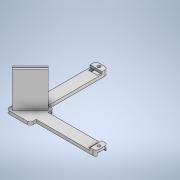
# Autodesk Inventor part: beamsplitter main
Saved by Autodesk Inventor 2022 (Build 260153000, 153)
## iProperties
Created: 2022-07-06
Part Number: beamsplitter main
Material: Generic
Document SubType Name: Modeling
Designer: Eli
Density: 1 g/cm^3
Appearance: Default
Author: Eli
Autodesk Inventor part; units mm, degrees
ref_plane "YZ Plane" through (0, 0, 0) normal (1, 0, 0) x (0, 1, 0)
ref_plane "XZ Plane" through (0, 0, 0) normal (0, 1, 0) x (-1, 0, 0)
sketch "Sketch1" plane through (0, 0, 0) normal (0, 1, 0) x (-1, 0, 0)
  line L0 (-6.35, 0) -> (-44.45, 0)
  line L1 (0, -44.45) -> (0, -6.35)
  line L2 (-38.1, -50.8) -> (-38.1, -171.45)
  line L3 (-31.75, -177.8) -> (-19.05, -177.8)
  line L4 (-12.7, -171.45) -> (-12.7, -50.8)
  line L5 (-25.4, 0) -> (-25.4, -50.8) construction
  line L6 (-44.45, -50.8) -> (-25.4, -50.8)
  line L7 (-12.7, -50.8) -> (-6.35, -50.8)
  line L8 (0, 0) -> (-50.8, -50.8) construction
  line L9 (-50.8, -38.1) -> (-171.45, -38.1)
  line L10 (-177.8, -31.75) -> (-177.8, -19.05)
  line L11 (-171.45, -12.7) -> (-50.8, -12.7)
  line L12 (-50.8, -6.35) -> (-50.8, -12.7)
  line L13 (-50.8, -38.1) -> (-50.8, -44.45)
  arc A0 (-50.8, -44.45) -> (-44.45, -50.8) centre (-44.45, -44.45) ccw
  arc A1 (-6.35, -50.8) -> (0, -44.45) centre (-6.35, -44.45) ccw
  arc A2 (0, -6.35) -> (-6.35, 0) centre (-6.35, -6.35) ccw
  arc A3 (-44.45, 0) -> (-50.8, -6.35) centre (-44.45, -6.35) ccw
  arc A4 (-19.05, -177.8) -> (-12.7, -171.45) centre (-19.05, -171.45) ccw
  arc A5 (-38.1, -171.45) -> (-31.75, -177.8) centre (-31.75, -171.45) ccw
  arc A6 (-171.45, -12.7) -> (-177.8, -19.05) centre (-171.45, -19.05) ccw
  arc A7 (-177.8, -31.75) -> (-171.45, -38.1) centre (-171.45, -31.75) ccw
  point P0 (-50.8, 0)
  point P1 (0, -50.8)
  point P2 (-38.1, -177.8)
  point P3 (-12.7, -177.8)
  point P4 (-177.8, -38.1)
  point P5 (-177.8, -12.7)
  dimension "d0" = 50.8
  dimension "d1" = 50.8
  dimension "d2" = 25.4
  dimension "d3" = 127
  dimension "d4" = 6.35
  dimension "d5" = 6.35
  dimension "d6" = 6.35
  constraints: 28 end point, 16 point on circle, 16 point on line, 16 tangent, 8 centre point, 5 equal radius, 5 parallel, 4 symmetric about line, 2 horizontal, 2 perpendicular, 1 midpoint, 1 vertical, 1 other
  measures "d0" distance of point (0, -50.8) L8.start
  measures "d1" distance of L8.start point (-50.8, 0)
  measures "d2" distance of point (-38.1, -177.8) point (-12.7, -177.8)
  measures "d3" distance of L2.start point (-38.1, -177.8)
  measures "d4" radius of A0
  measures "d5" radius of A1
  measures "d6" radius of A4
extrude "Extrusion2" add sketch "Sketch1" along normal blind 6.35
sketch "Sketch2" plane through (0, 6.35, 0) normal (0, 1, 0) x (1, 0, 0)
  arc A0 (50.8, 44.45) -> (44.45, 50.8) centre (44.45, 44.45) ccw construction
  arc A1 (0, 6.35) -> (6.35, 0) centre (6.35, 6.35) ccw construction
  line L0 (44.45, 44.45) -> (6.35, 6.35) construction
  line L1 (6.6306, 6.0694) -> (44.7306, 44.1694)
  line L2 (6.6306, 6.0694) -> (9.1706, 3.5294)
  line L3 (9.1706, 3.5294) -> (47.2706, 41.6294)
  line L4 (44.7306, 44.1694) -> (47.2706, 41.6294)
  line L5 (6.0694, 6.6306) -> (44.1694, 44.7306)
  line L6 (6.0694, 6.6306) -> (3.5294, 9.1706)
  line L7 (3.5294, 9.1706) -> (41.6294, 47.2706)
  line L8 (44.1694, 44.7306) -> (41.6294, 47.2706)
  point P0 (0, 0)
  dimension "d14" = 38.1
  dimension "d15" = 0.3969
  dimension "d16" = 0.2806
  dimension "d17" = 90
  dimension "d18" = 2.54
  constraints: 18 end point, 4 symmetric about line, 3 parallel
  measures "d14" horizontal distance of L1.start L1.end
  measures "d15" distance between parallel lines of L0 L1
  measures "d16" horizontal distance of L0.end L1.start
  measures "d17" angle of L2 L1
  measures "d18" horizontal distance of L1.start L2.end
extrude "Extrusion3" add sketch "Sketch2" along normal blind 76.2
sketch "Sketch3" plane through (0, 6.35, 0) normal (0, 1, 0) x (1, 0, 0)
  line L0 (6.0694, 6.6306) -> (44.1694, 44.7306) projected
  line L1 (47.2706, 41.6294) -> (44.7306, 44.1694) projected
  line L2 (44.1694, 44.7306) -> (44.7306, 44.1694)
  line L3 (44.7306, 44.1694) -> (6.6306, 6.0694) projected
  line L4 (44.7306, 44.1694) -> (6.6306, 6.0694)
  line L5 (6.0694, 6.6306) -> (3.5294, 9.1706) projected
  line L6 (6.6306, 6.0694) -> (6.0694, 6.6306)
  line L7 (6.0694, 6.6306) -> (44.1694, 44.7306)
  point P0 (0, 0)
  constraints: 8 end point, 3 perpendicular, 1 collinear
extrude "Extrusion4" add sketch "Sketch3" along normal blind 50.8
sketch "Sketch4" plane through (0, 6.35, 0) normal (0, 1, 0) x (1, 0, 0)
  arc A0 (19.05, 177.8) -> (12.7, 171.45) centre (19.05, 171.45) ccw construction
  arc A1 (38.1, 171.45) -> (31.75, 177.8) centre (31.75, 171.45) ccw construction
  line L0 (19.05, 171.45) -> (31.75, 171.45) construction
  circle A2 centre (25.4, 171.45) radius 3.1386
  line L1 (12.7, 171.45) -> (12.7, 50.8) projected
  line L2 (12.7, 165.1) -> (38.1, 165.1)
  line L3 (38.1, 165.1) -> (38.1, 171.45)
  line L4 (12.7, 165.1) -> (12.7, 171.45)
  line L5 (31.75, 177.8) -> (19.05, 177.8) projected
  line L6 (19.05, 177.8) -> (31.75, 177.8)
  arc A3 (19.05, 177.8) -> (12.7, 171.45) centre (19.05, 171.45) ccw
  arc A4 (38.1, 171.45) -> (31.75, 177.8) centre (31.75, 171.45) ccw
  point P0 (0, 0)
  point P1 (14.5599, 175.9401)
  dimension "d23" = 6.2773
  dimension "d68" = 6.35
  constraints: 10 end point, 5 point on circle, 3 centre point, 3 point on line, 2 concentric, 2 horizontal, 1 coincident, 1 collinear, 1 midpoint, 1 perpendicular, 1 other
  measures "d23" diameter of A2
  measures "d68" distance between parallel lines of L0 L2
ref_plane "Work Plane1" through (48.9401, 6.35, -48.9401) normal (-0.7071, 0, -0.7071) x (0, -1, 0)
extrude "Extrusion6" add sketch "Sketch4" along normal blind 5.08
sketch "Sketch11" plane through (0, 0, 0) normal (0, -1, 0) x (1, 0, 0)
  line L0 (34.925, -177.8) -> (15.875, -177.8) construction
  line L1 (25.4, -177.8) -> (25.4, -169.6336) construction
  line L2 (34.925, -177.8) -> (15.875, -177.8)
  line L3 (15.875, -177.8) -> (15.875, -158.75)
  line L4 (15.875, -158.75) -> (34.925, -158.75)
  line L5 (34.925, -158.75) -> (34.925, -177.8)
  line L6 (31.75, -177.8) -> (19.05, -177.8) projected
  point P0 (0, 0)
  dimension "d71" = 19.05
  dimension "d74" = 19.05
  constraints: 12 end point, 3 midpoint, 2 parallel, 1 collinear, 1 horizontal, 1 perpendicular, 1 vertical, 1 other
  measures "d71" distance of L4.end L0.start
  measures "d74" distance of L3.end L4.end
extrude "Extrusion7" cut sketch "Sketch11" against normal blind 6.35
mirror "Mirror2" about plane through (48.9401, 6.35, -48.9401) normal (-0.7071, 0, -0.7071) of "Extrusion6", "Extrusion7"
equation "\"d37\" = 55deg"
equation "\"Sketch5_Pitch\" = 1.27"
equation "\"d56\" = 55deg"
equation "\"Sketch8_Pitch\" = 1.27"
body "Solid2"
